Keyboard (Autodesk Fusion 360 design; units mm, degrees)
Autodesk Fusion 360 part; units mm, degrees
sketch "Sketch1" plane through (0, 0, 0) normal (0, 1, 0) x (1, 0, 0)
  line L0 (50.9028, -9.9887) -> (-55.575, -24.7971)
  line L1 (-68.1287, -14.808) -> (-68.1287, 13.8249)
  line L2 (51.6419, 24.9918) -> (-57.2166, 24.9918)
  spline S0 degree 5 poles (50.9028, -9.9887) (51.2119, -9.9351) (51.8302, -9.8158) (52.7581, -9.6007) (53.996, -9.2414) (55.543, -8.6696) (57.0845, -7.9717) (58.6109, -7.1413) (60.1052, -6.1691) (61.5427, -5.042) (62.8931, -3.7475) (64.1232, -2.2775) (65.1988, -0.6323) (66.0873, 1.1761) (66.7603, 3.1184) (67.1954, 5.1516) (67.3783, 7.2252) (67.3045, 9.286) (66.9817, 11.2845) (66.432, 13.1798) (65.6943, 14.946) (64.818, 16.5693) (63.8539, 18.0452) (62.8465, 19.3746) (61.8264, 20.5611) (60.8001, 21.6073) (59.7523, 22.5139) (58.6565, 23.281) (57.4827, 23.9081) (56.2071, 24.3954) (54.8168, 24.7436) (53.608, 24.9115) (52.6463, 24.9757) (51.9807, 24.991) (51.6419, 24.9918) knots 0 0 0 0 0 0 0.033333 0.066667 0.1 0.133333 0.166667 0.2 0.233333 0.266667 0.3 0.333333 0.366667 0.4 0.433333 0.466667 0.5 0.533333 0.566667 0.6 0.633333 0.666667 0.7 0.733333 0.766667 0.8 0.833333 0.866667 0.9 0.933333 0.966667 1 1 1 1 1 1
  spline S1 degree 5 poles (-55.575, -24.7971) (-56.0802, -24.8501) (-57.0686, -24.9344) (-58.4857, -24.9956) (-60.242, -24.9448) (-62.2, -24.6449) (-63.8982, -24.0867) (-65.3136, -23.247) (-66.4305, -22.1104) (-67.2563, -20.684) (-67.8109, -18.9879) (-68.0547, -17.432) (-68.132, -16.1601) (-68.1375, -15.2664) (-68.1287, -14.808) knots 0 0 0 0 0 0 0.1 0.2 0.3 0.4 0.5 0.6 0.7 0.8 0.9 1 1 1 1 1 1
  spline S2 degree 5 poles (-57.2166, 24.9918) (-57.669, 24.9969) (-58.5534, 24.987) (-59.8187, 24.9125) (-61.3809, 24.6914) (-63.1118, 24.1986) (-64.6008, 23.4699) (-65.8283, 22.4861) (-66.7834, 21.2367) (-67.4769, 19.7321) (-67.9284, 17.9915) (-68.112, 16.4258) (-68.1562, 15.1603) (-68.1447, 14.2767) (-68.1287, 13.8249) knots 0 0 0 0 0 0 0.1 0.2 0.3 0.4 0.5 0.6 0.7 0.8 0.9 1 1 1 1 1 1
  point P0 (58.398, -7.2268)
  point P1 (65.4258, -0.0892)
  point P2 (66.8661, 11.5139)
  point P3 (62.4418, 19.8251)
  point P4 (57.9224, 23.6482)
  point P5 (-65.4504, -23.0005)
  point P6 (-65.7619, 22.4183)
  constraint vertical L1
  constraint perpendicular L1 L2
extrude "Extrude1" add sketch "Sketch1" along normal blind 305
sketch "Sketch2" plane through (2.3287, 0, 16.7441) normal (0.137749, 0, 0.990467) x (0, 1, 0)
  line L0 (0, 58.461) -> (0, -49.0416)
  line L1 (0, -49.0416) -> (305, -49.0416)
  line L2 (305, -49.0416) -> (305, 58.461)
  line L3 (305, 58.461) -> (0, 58.461)
  line L4 (10.3, 54.911) -> (294.7, 54.911)
  line L5 (297.7, 51.911) -> (297.7, -42.489)
  line L6 (294.7, -45.489) -> (10.3, -45.489)
  line L7 (7.3, -42.489) -> (7.3, 51.911)
  arc A0 (294.7, -45.489) -> (297.7, -42.489) centre (294.7, -42.489) ccw
  arc A1 (297.7, 51.911) -> (294.7, 54.911) centre (294.7, 51.911) ccw
  arc A2 (10.3, 54.911) -> (7.3, 51.911) centre (10.3, 51.911) ccw
  arc A3 (7.3, -42.489) -> (10.3, -45.489) centre (10.3, -42.489) ccw
  point P0 (7.3, 54.911)
  point P1 (297.7, 54.911)
  point P2 (7.3, -45.489)
  dimension "d21" = 290.4
  dimension "d22" = 100.4
  dimension "d24" = 7.3
  dimension "d25" = 3.55
  dimension "d26" = 3
  constraint horizontal L4
  constraint vertical L5
  constraint horizontal L6
  constraint vertical L7
  constraint tangent L5 A0
  constraint tangent L6 A0
  constraint coincident P1 L4
  constraint coincident P1 L5
  constraint tangent L4 A1
  constraint tangent L5 A1
  constraint equal A0 A1
  constraint coincident P0 L4
  constraint coincident P0 L7
  constraint tangent L4 A2
  constraint tangent L7 A2
  constraint equal A0 A2
  constraint coincident P2 L6
  constraint coincident P2 L7
  constraint tangent L6 A3
  constraint tangent L7 A3
  constraint equal A0 A3
  measures "d21" distance of P0 P1
  measures "d22" distance of P0 P2
  measures "d24" distance of L0 L7
  measures "d25" distance of L3 L4
  measures "d26" radius of A0
extrude "Extrude5" cut sketch "Sketch2" against normal blind 27 contours L4 L5 L6 L7 A0 A1 A2 A3
fillet "Fillet1" radius 3 6 edges at (-2.3361, 305, 17.3929) (-65.2392, 305, 23.173) (-68.1287, 305, 0.4915) (-65.7604, 305, -22.4199) (-2.7874, 305, -24.9918) (67.2423, 305, -9.2705)
fillet "Fillet2" radius 3 6 edges at (-2.3361, 0, 17.3929) (-65.2392, 0, 23.173) (-68.1287, 0, 0.4915) (-65.7604, 0, -22.4199) (-2.7874, 0, -24.9918) (67.2423, 0, -9.2705)
sketch "Sketch6" plane through (-54.3876, 0, 7.564) normal (0.990467, 0, -0.137749) x (0, 1, 0)
  line L0 (294.7, 16.9053) -> (10.3, 16.9053)
  line L1 (10.3, 16.9053) -> (10.3, -10.0947)
  line L2 (10.3, -10.0947) -> (294.7, -10.0947)
  line L3 (294.7, -10.0947) -> (294.7, 16.9053)
  line L4 (135.3, 9.9053) -> (149.3, 9.9053)
  line L5 (149.3, 9.9053) -> (149.3, -2.0947)
  line L6 (149.3, -2.0947) -> (135.3, -2.0947)
  line L7 (135.3, -2.0947) -> (135.3, 9.9053)
  line L8 (152.5, 16.9053) -> (152.5, -10.0947) construction
  dimension "d43" = 14
  dimension "d44" = 12
  dimension "d45" = 125
  dimension "d46" = 142.2
  dimension "d47" = 7
  constraint horizontal L4
  constraint vertical L5
  constraint horizontal L6
  constraint vertical L7
  constraint coincident L0 L8.start
  constraint coincident L2 L8.end
  constraint perpendicular L2 L8
  measures "d43" distance of L4.start L4.end
  measures "d44" distance of L4.start L6.end
  measures "d45" distance of L1 L7
  measures "d46" distance of L3 L8
  measures "d47" distance of L0 L4
extrude "Extrude8" cut sketch "Sketch6" against normal blind 20 contours L4 L5 L6 L7
